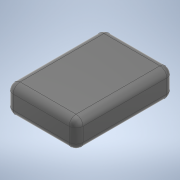
# Autodesk Inventor part: Battery Pack
Saved by Autodesk Inventor 2021 (Build 250183000, 183)
## iProperties
Created: 2020-07-18
Part Number: Battery Pack
Material: Generic
Document SubType Name: Modeling
Designer: Andrew
Density: 1 g/cm^3
Appearance: Default
Author: Andrew
Autodesk Inventor part; units mm, degrees
ref_plane "YZ Plane" through (0, 0, 0) normal (1, 0, 0) x (0, 1, 0)
ref_plane "XZ Plane" through (0, 0, 0) normal (0, 1, 0) x (-1, 0, 0)
ref_plane "XY Plane" through (0, 0, 0) normal (0, 0, 1) x (1, 0, 0)
sketch "Sketch1" plane through (0, 0, 0) normal (0, 1, 0) x (-1, 0, 0)
  line L0 (0, 0) -> (50, 0)
  line L1 (50, 0) -> (50, -70)
  line L2 (50, -70) -> (0, -70)
  line L3 (0, -70) -> (0, 0)
  dimension "d0" = 50
  dimension "d1" = 70
  constraints: 8 end point, 2 parallel, 1 horizontal, 1 perpendicular
  measures "d0" distance of L1.end L2.end
  measures "d1" distance of L0.end L1.end
extrude "Extrusion1" add sketch "Sketch1" along normal blind 20
fillet "Fillet2" radius 5 12 edges at (-25, 20, -70) (0, 20, -35) (-50, 20, -35) (-25, 20, 0) (0, 10, -70) (0, 10, 0) (0, 0, -35) (-25, 0, -70) (-50, 10, -70) (-50, 0, -35) (-50, 10, 0) (-25, 0, 0)
body "Solid1"
